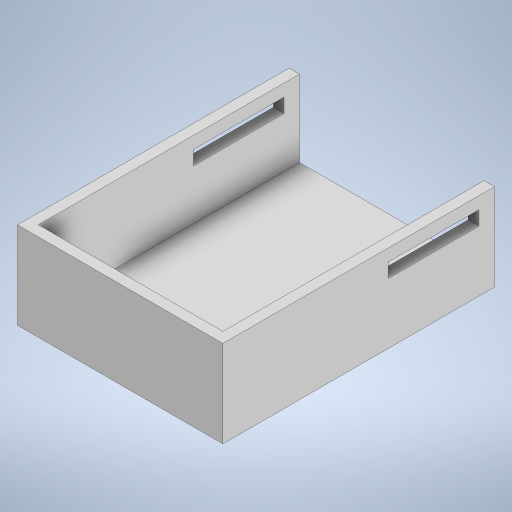
# Autodesk Inventor part: arduino array box v03
Saved by Autodesk Inventor 2023 (Build 270158000, 158)
## iProperties
Created: 2024-07-12
Part Number: arduino array box v03
Material: Generic
Document SubType Name: Modeling
Designer: Akramilab
Density: 1 g/cm^3
Appearance: Default
Author: Akramilab
Autodesk Inventor part; units mm, degrees
ref_plane "YZ Plane" through (0, 0, 0) normal (1, 0, 0) x (0, 1, 0)
ref_plane "XZ Plane" through (0, 0, 0) normal (0, 1, 0) x (-1, 0, 0)
ref_plane "XY Plane" through (0, 0, 0) normal (0, 0, 1) x (1, 0, 0)
sketch "Sketch2" plane through (0, 0, 0) normal (0, 1, 0) x (-1, 0, 0)
  line L0 (0, 0) -> (-59, 0)
  line L1 (-59, 0) -> (-59, 78)
  line L2 (-59, 78) -> (0, 78)
  line L3 (0, 78) -> (0, 0)
  dimension "d0" = 59
  dimension "d1" = 78
  constraints: 8 end point, 2 parallel, 1 horizontal, 1 perpendicular
  measures "d0" distance of L0.start L0.end
  measures "d1" distance between parallel lines of L2 L0
extrude "Extrusion1" add sketch "Sketch2" along normal blind 25
shell "Shell1" thickness 3 removed faces 1 at (39.3333, 25, 52)
sketch "Sketch4" plane through (59, 0, 0) normal (0, 0, -1) x (-1, 0, 0)
  point P0 (59, 0)
sketch "Sketch5" plane through (3, 3, 3) normal (0, 0, 1) x (1, 0, 0)
  line L0 (0, 0) -> (0, 22) projected
  line L1 (0, 22) -> (53, 22) projected
  line L2 (0, 0) -> (53, 0)
  line L3 (53, 0) -> (53, 22)
  line L4 (53, 22) -> (0, 22)
  line L5 (0, 22) -> (0, 0)
  point P0 (-3, -3)
  constraints: 8 end point, 2 parallel, 1 horizontal, 1 perpendicular
extrude "Extrusion3" cut sketch "Sketch5" against normal blind 10
sketch "Sketch6" plane through (0, 0, 0) normal (-1, 0, 0) x (0, 0, 1)
  line L0 (4.5, 21.5) -> (30.5, 21.5)
  line L1 (30.5, 21.5) -> (30.5, 17.5)
  line L2 (30.5, 17.5) -> (4.5, 17.5)
  line L3 (4.5, 17.5) -> (4.5, 21.5)
  line L4 (0, 0) -> (0, 25) projected
  line L5 (0, 0) -> (78, 0) projected
  dimension "d19" = 26
  dimension "d20" = 4
  dimension "d21" = 4.5
  dimension "d22" = 17.5
  constraints: 8 end point, 2 parallel, 1 horizontal, 1 perpendicular
  measures "d19" distance of L0.start L0.end
  measures "d20" distance of L2.end L0.start
  measures "d21" distance between parallel lines of L4 L3
  measures "d22" distance between parallel lines of L2 L5
extrude "Extrusion4" cut sketch "Sketch6" against normal through all
body "Solid1"
